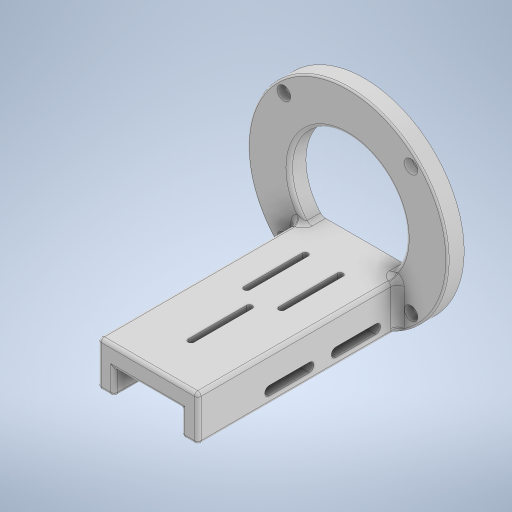
# Autodesk Inventor part: Drzak_svetlo_VMR_11566W_v2
Saved by Autodesk Inventor 2023 (Build 270158000, 158)
## iProperties
Created: 2025-01-06
Part Number: Drzak_svetlo_VMR_11566W_v2
Material: Všeobecné
Document SubType Name: Modeling
Designer: lisnik
Density: 1 g/cm^3
Appearance: Výchozí
Author: lisnik
Autodesk Inventor part; units mm, degrees
ref_plane "YZ Plane" through (0, 0, 0) normal (1, 0, 0) x (0, 1, 0)
ref_plane "XZ Plane" through (0, 0, 0) normal (0, 1, 0) x (-1, 0, 0)
ref_plane "XY Plane" through (0, 0, 0) normal (0, 0, 1) x (1, 0, 0)
sketch "Náčrt1" plane through (0, 0, 0) normal (0, 0, 1) x (1, 0, 0)
  line L0 (-84, 0) -> (84, 0) projected
  line L1 (0, -84) -> (0, 84) projected
  circle A0 centre (0, 0) radius 60
  circle A1 centre (0, 0) radius 35
  dimension "d0" = 120
  dimension "d1" = 70
  constraints: 2 centre point, 2 coincident
  measures "d0" diameter of A0
  measures "d1" diameter of A1
extrude "Vysunutí1" add sketch "Náčrt1" along normal blind 10 contours A1 L1 A0 L0 | L0 A0 L1 A1 | A1 L0 A0 L1 | L1 A0 L0 A1
sketch "Náčrt2" plane through (0, 0, 10) normal (0, 0, 1) x (1, 0, 0)
  line L0 (-84, 0) -> (84, 0) projected
  line L1 (0, -84) -> (0, 84) projected
  line L2 (0, 0) -> (-42.4264, 42.4264) construction
  circle A0 centre (0, 0) radius 60 projected
  point P0 (-38.1838, 38.1838)
  dimension "d4" = 45
  dimension "d5" = 54
  constraints: 2 end point, 1 point on line, 2 other
  measures "d4" angle of L1 L2
  measures "d5" distance of L2.start point (-38.184, 38.184)
hole "Díra1" at (-38.1838, 38.1838, 10) direction (0, 0, -1) diameter 4.5 end through all counterbore diameter 8 counterbore depth 4.6 clearance for "Šroub s hlavou s vnitřním vybráním ISO 4762" size "M4" standard "ISO"
pattern_circular "Kruhové pole1" count 4 over 360 about axis through (0, 0, -10) along (0, 0, 1) of "Díra1"
sketch "Náčrt3" plane through (0, 0, 10) normal (0, 0, 1) x (1, 0, 0)
  line L0 (0, -90) -> (0, 85) projected
  line L1 (-84, 0) -> (84, 0) projected
  circle A0 centre (0, 0) radius 60 projected
  line L2 (-30, -51.5) -> (30, -51.5)
  line L3 (30, -51.5) -> (30, -24.5)
  line L4 (30, -24.5) -> (-30, -24.5)
  line L5 (-30, -24.5) -> (-30, -51.5)
  circle A1 centre (0, 0) radius 35 projected
  line L6 (-20.2, -51.5) -> (20.2, -51.5)
  line L7 (20.2, -51.5) -> (20.2, -36.5)
  line L8 (20.2, -36.5) -> (-20.2, -36.5)
  line L9 (-20.2, -36.5) -> (-20.2, -51.5)
  point P0 (0, -36.5)
  dimension "d17" = 60
  dimension "d20" = 27
  dimension "d21" = 12
  dimension "d22" = 9.8
  dimension "d75" = 24.5
  dimension "d76" = 9.8
  constraints: 16 end point, 4 parallel, 2 horizontal, 2 perpendicular, 2 point on line, 1 midpoint
  measures "d17" distance of L2.start L2.end
  measures "d20" distance of L2.end L3.end
  measures "d21" distance between parallel lines of L8 L4
  measures "d22" distance between parallel lines of L3 L7
  measures "d75" distance between parallel lines of L4 L1
  measures "d76" distance between parallel lines of L5 L9
extrude "Vysunutí2" add sketch "Náčrt3" along normal blind 120 and the other way blind 10 contours L8 L9 L2 L5 L4 A1 L0 | L0 A1 L4 L3 L2 L7 L8 | A1 L4 L0 | L0 L4 A1
sketch "Náčrt5" plane through (24.995, -24.5, 10) normal (0, 1, 0) x (1, 0, 0)
  circle A0 centre (-35.495, -15) radius 1.75
  circle A1 centre (-14.495, -15) radius 1.75
  circle A2 centre (-24.995, -59) radius 1.75
  line L0 (-24.995, 36) -> (-24.995, -146) projected
  line L1 (-54.995, 0) -> (0, 0) projected
  circle A3 centre (-14.495, -50) radius 1.75
  circle A4 centre (-24.995, -94) radius 1.75
  line L2 (-14.495, -15) -> (-35.495, -15) construction
  line L3 (-35.495, -15) -> (-35.495, -50) construction
  line L4 (-35.495, -50) -> (-14.495, -50) construction
  line L5 (-14.495, -50) -> (-14.495, -15) construction
  circle A5 centre (-35.495, -50) radius 1.75
  line L6 (-37.245, -50) -> (-37.245, -15)
  line L7 (-33.745, -50) -> (-33.745, -15)
  line L8 (-16.245, -50) -> (-16.245, -15)
  line L9 (-12.745, -50) -> (-12.745, -15)
  circle A6 centre (-14.495, -50) radius 4.75
  line L10 (-19.245, -50) -> (-19.245, -15)
  line L11 (-9.745, -50) -> (-9.745, -15)
  circle A7 centre (-14.495, -15) radius 4.75
  line L12 (-30.745, -50) -> (-30.745, -15)
  circle A8 centre (-35.495, -50) radius 4.75
  line L13 (-40.245, -50) -> (-40.245, -15)
  circle A9 centre (-35.495, -15) radius 4.75
  circle A10 centre (-24.995, -94) radius 4.75
  circle A11 centre (-24.995, -59) radius 4.75
  line L14 (-29.745, -94) -> (-20.245, -94)
  line L15 (-20.245, -94) -> (-20.245, -59)
  line L16 (-20.245, -59) -> (-29.745, -59)
  line L17 (-29.745, -59) -> (-29.745, -94)
  line L18 (-26.745, -94) -> (-23.245, -94)
  line L19 (-23.245, -94) -> (-23.245, -59)
  line L20 (-23.245, -59) -> (-26.745, -59)
  line L21 (-26.745, -59) -> (-26.745, -94)
  point P0 (-24.995, 10)
  point P1 (-23.245, -59)
  point P2 (-26.745, -59)
  point P3 (-9.745, -55)
  point P4 (-9.745, -20)
  point P5 (-19.245, -20)
  point P6 (-19.245, -55)
  point P7 (-37.245, -19.4159)
  point P8 (-33.745, -19.4159)
  point P9 (-30.745, -20)
  point P10 (-40.245, -20)
  point P11 (-20.245, -94)
  point P12 (-29.745, -59)
  point P13 (-37.245, -45.5841)
  point P14 (-33.745, -45.5841)
  point P15 (-16.245, -19.4159)
  point P16 (-16.245, -45.5841)
  point P17 (-12.745, -19.4159)
  point P18 (-12.745, -45.5841)
  dimension "d46" = 3
  dimension "d25" = 3.5
  dimension "d26" = 3.5
  dimension "d27" = 3.5
  dimension "d28" = 21
  dimension "d29" = 10.5
  dimension "d30" = 44
  dimension "d31" = 15
  dimension "d32" = 44
  dimension "d36" = 35
  dimension "d37" = 3
  dimension "d38" = 3
  dimension "d39" = 3
  dimension "d40" = 3
  dimension "d41" = 3
  dimension "d42" = 3
  dimension "d43" = 3
  dimension "d44" = 3
  dimension "d45" = 35
  dimension "d47" = 3
  constraints: 40 end point, 12 point on circle, 11 parallel, 9 centre point, 6 point on line, 4 midpoint, 4 tangent, 3 horizontal, 3 perpendicular, 2 coincident, 2 equal radius, 1 vertical, 13 other
  measures "d25" diameter of A0
  measures "d26" diameter of A1
  measures "d27" diameter of A2
  measures "d28" distance of A0.centre L2.start
  measures "d29" horizontal distance of A2.centre A0.centre
  measures "d30" vertical distance of A2.centre A0.centre
  measures "d31" distance from line of L1 A0.centre
  measures "d32" vertical distance of A2.centre L2.start
  measures "d36" distance between parallel lines of L2 L4
  measures "d37" radial gap between concentric circles of A3 A6
  measures "d38" distance between parallel lines of L8 L10
  measures "d39" distance between parallel lines of L9 L11
  measures "d40" radial gap between concentric circles of A1 A7
  measures "d41" distance between parallel lines of L7 L12
  measures "d42" radial gap between concentric circles of A5 A8
  measures "d43" distance between parallel lines of L6 L13
  measures "d44" radial gap between concentric circles of A0 A9
  measures "d45" distance of point (-24.995, -94) A2.centre
extrude "Vysunutí4" cut sketch "Náčrt5" against normal through all contours A0 | L7 A9 L6 A0 | L7 A8 L6 A9 | L7 A5 L6 A8 | A5 | A1 | L9 A7 L8 A1 | L9 A6 L8 A7 | L9 A3 L8 A6 | A3 | L16 L0 A2 | L19 A11 L0 A2 | A2 L0 L16 | L0 L16 A2 | L0 A11 L21 A2 | A2 L16 L0 | L19 A10 L0 A11 | L0 A10 L21 A11 | L19 A4 L0 A10 | L0 A4 L21 A10 | L14 L0 A4 | A4 L0 L14 | L0 L14 A4 | A4 L14 L0 picked at (-34.4079, -18.5726) picked at (-36.5821, -46.4274) picked at (-15.5821, -18.5726) picked at (-15.5821, -46.4274)
extrude "Vysunutí5" cut sketch "Náčrt5" along normal blind 5 from surface at -12 contours A0 | L7 A9 L6 A0 | A0 L6 A9 L7 | A9 L12 A8 L7 | L6 A8 L13 A9 | A8 L6 A5 L7 | L7 A5 L6 A8 | A5 | A1 | L9 A7 L8 A1 | A1 L8 A7 L9 | A7 L11 A6 L9 | L8 A6 L10 A7 | A6 L8 A3 L9 | L9 A3 L8 A6 | A3 | A2 L0 A11 L16 | L16 A11 L19 | A2 L16 A11 L0 | L15 A10 L19 A11 | L21 A11 L16 | L14 L19 A10 | A10 L0 A4 L14 | A11 L21 A10 L17 | A10 L14 A4 L0 | A10 L21 L14
fillet "Zaoblení4" radius 2 8 edges at (30, -38, 130) (0, -24.5, 130) (-30, -38, 130) (-25.1, -51.5, 130) (-20.2, -44, 130) (0, -36.5, 130) (20.2, -44, 130) (25.1, -51.5, 130)
fillet "Zaoblení5" radius 2 13 edges at (29.4142, -50.9142, 129.4142) (30, -51.5, 69) (20.7858, -50.9142, 129.4142) (20.2, -51.5, 69) (-20.7858, -50.9142, 129.4142) (-20.2, -51.5, 69) (-29.4142, -50.9142, 129.4142) (-30, -51.5, 69) (29.4142, -25.0858, 129.4142) (30, -24.5, 69) (-29.4142, -25.0858, 129.4142) (-30, -24.5, 69) (0, 35, 10)
fillet "Zaoblení6" radius 1 5 edges at (-20.7858, -35.9142, 129.4142) (-20.2, -36.5, 69) (20.7858, -35.9142, 129.4142) (20.2, -36.5, 69) (-60, 0, 10)
fillet "Zaoblení7" radius 4 21 edges at (29.4142, -50.9142, 10) (25.1, -51.5, 10) (20.7858, -50.9142, 10) (20.2, -43.5, 10) (19.9071, -36.7929, 10) (0, -36.5, 10) (-19.9071, -36.7929, 10) (-20.2, -43.5, 10) (-20.7858, -50.9142, 10) (-25.1, -51.5, 10) (-29.4142, -50.9142, 10) (-30, -38, 10) (-29.4142, -25.0858, 10) (-27.8632, -24.5, 10) (-25.9296, -24.5, 9.4967) (-24.995, -24.5, 4) (29.4142, -25.0858, 10) (27.8632, -24.5, 10) (25.9296, -24.5, 9.4967) (24.995, -24.5, 4) (30, -38, 10)
sketch "Náčrt9" plane through (30, -49.5, 128) normal (1, 0, 0) x (0, 0, -1)
  line L0 (0, -2) -> (115.1277, -2) projected
  line L1 (118, 1.2817) -> (118, 108.5) projected
  line L2 (128, 109.5) -> (128, -10.5) projected
  point P0 (128, 49.5)
  point P1 (93, 5.5)
  point P2 (53, 5.5)
  dimension "d80" = 7.5
  dimension "d81" = 7.5
  dimension "d82" = 40
  dimension "d84" = 35
  measures "d80" distance from line of L0 point (93, 5.5)
  measures "d81" distance from line of L0 point (53, 5.5)
  measures "d82" distance of point (93, 5.5) point (53, 5.5)
  measures "d84" distance from line of L2 point (93, 5.5)
hole "Díra3" at (30, -44, 75) at (30, -44, 35) direction (-1, 0, 0) diameter 5.5 end through all clearance for "Strojní šroub se zápustnou hlavou" size "M5" standard "Ansi M metrický profil"
sketch "Náčrt10" plane through (30, -49.5, 128) normal (1, 0, 0) x (0, 0, -1)
  circle A0 centre (53, 5.5) radius 2.75 projected
  circle A1 centre (93, 5.5) radius 2.75 projected
  line L0 (81, 5.5) -> (105, 5.5) construction
  line L1 (81, 2.75) -> (105, 2.75)
  line L2 (105, 8.25) -> (81, 8.25)
  arc A2 (81, 8.25) -> (81, 2.75) centre (81, 5.5) ccw
  arc A3 (105, 2.75) -> (105, 8.25) centre (105, 5.5) ccw
  line L3 (41, 5.5) -> (65, 5.5) construction
  line L4 (41, 2.75) -> (65, 2.75)
  line L5 (65, 8.25) -> (41, 8.25)
  arc A4 (41, 8.25) -> (41, 2.75) centre (41, 5.5) ccw
  arc A5 (65, 2.75) -> (65, 8.25) centre (65, 5.5) ccw
  point P0 (128, 49.5)
  point P1 (93, 2.75)
  point P2 (93, 8.25)
  dimension "d92" = 12
  dimension "d94" = 12
  constraints: 16 end point, 8 point on circle, 8 tangent, 4 centre point, 2 equal radius, 2 horizontal, 2 midpoint, 2 parallel
  measures "d92" distance of A1.centre L0.end
  measures "d94" distance of A0.centre L3.end
extrude "Vysunutí7" cut sketch "Náčrt10" against normal through all contours A0 | A0 L5 A5 L4 | A0 L4 A4 L5 | A1 L2 A3 L1 | A1 L1 A2 L2
sketch "Náčrt11" plane through (0, 0, 0) normal (0, 0, -1) x (-1, 0, 0)
  circle A0 centre (-38.1838, -38.1838) radius 2.25 projected
  circle A1 centre (38.1838, -38.1838) radius 2.25 projected
  circle A2 centre (0, 0) radius 60 projected
  circle A3 centre (38.1838, 38.1838) radius 2.25 projected
  circle A4 centre (-38.1838, 38.1838) radius 2.25 projected
  arc A5 (23.254, -24.5) -> (26.2546, -23.1452) centre (23.254, -20.5) ccw projected
  line L0 (23.254, -24.5) -> (-23.254, -24.5) projected
  arc A6 (-26.2546, -23.1452) -> (-23.254, -24.5) centre (-23.254, -20.5) ccw projected
  arc A7 (26.2546, -23.1452) -> (-26.2546, -23.1452) centre (0, 0) ccw projected
  circle A8 centre (0, 0) radius 60 projected
  circle A9 centre (0, -60) radius 2.5
  line L1 (84, 0) -> (-84, 0) projected
  line L2 (0, -86.2897) -> (0, 84.3816) projected
  dimension "d97" = 5
  constraints: 1 centre point, 1 point on line, 1 vertical alignment, 1 other
  measures "d97" diameter of A9
extrude "Vysunutí8" cut sketch "Náčrt11" against normal through all contours A9 L2 A2 | A2 L2 A9 | L2 A9 A2 | A2 A9 L2
